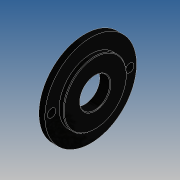
# Autodesk Inventor part: P120RondelleAppui
Saved by Autodesk Inventor 2015 SP1 (Build 190203100, 203)
## iProperties
Created: 2017-01-12
Part Number: P120RondelleAppui
Material: ABS Plastic
Document SubType Name: Modeling
Designer: serge.amoos
Density: 1.06 g/cm^3
Appearance: Smooth - Black
Author: serge.amoos
Autodesk Inventor part; units mm, degrees
ref_plane "YZ Plane" through (0, 0, 0) normal (1, 0, 0) x (0, 1, 0)
ref_plane "XZ Plane" through (0, 0, 0) normal (0, 1, 0) x (-1, 0, 0)
ref_plane "XY Plane" through (0, 0, 0) normal (0, 0, 1) x (1, 0, 0)
sketch "Sketch1" plane through (0, 0, 0) normal (0, 0, 1) x (1, 0, 0)
  line L0 (-4.2, 0) -> (0.7, 0) construction
  line L1 (0, -3.05) -> (0, 18.3) construction
  line L2 (0, 5) -> (-3.5, 5)
  line L3 (-3.5, 5) -> (-3.5, 15.25)
  line L4 (-3.5, 15.25) -> (-1.5, 15.25)
  line L5 (-1.5, 15.25) -> (-1.5, 10.5)
  line L6 (-1.5, 10.5) -> (0, 10.5)
  line L7 (0, 10.5) -> (0, 5)
  point P0 (0, 0)
  dimension "d0" = 10
  dimension "d1" = 21
  dimension "d2" = 1.5
  dimension "d3" = 2
  dimension "d4" = 30.5
  constraints: 12 end point, 4 perpendicular, 2 point on line, 1 collinear, 1 horizontal
  measures "d0" diameter of L2 L0
  measures "d1" diameter of L6 L0
  measures "d2" distance between parallel lines of L1 L5
  measures "d3" distance between parallel lines of L5 L3
  measures "d4" diameter of L4 L0
revolve "Revolution1" add sketch "Sketch1" angle 360 about axis through (-10, 0, 0) along (1, 0, 0)
sketch "Sketch2" plane through (-3.5, 0, 0) normal (-1, 0, 0) x (0, 0, 1)
  line L0 (0, -21.35) -> (0, 21.35) projected
  line L1 (-21.35, 0) -> (21.35, 0) projected
  point P0 (0, 0)
  point P1 (0, 13)
  dimension "d6" = 13
  constraints: 1 point on line
  measures "d6" distance from line of L1 point (0, 13)
hole "Hole1" at (-3.5, 13, 0) direction (1, 0, 0) diameter 2.8 end through all
mirror "Mirror1" about plane through (0, 0, 0) normal (0, 1, 0) of "Hole1"
fillet "Fillet1" radius 0.2 2 edges at (0, -10.5, 0) (0, -5, 0)
body "Solid1"
